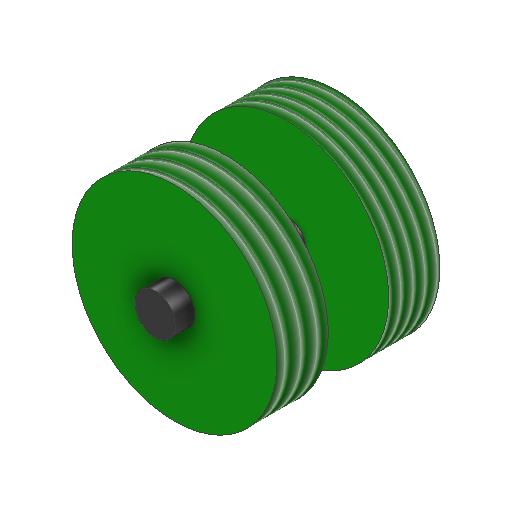
# Autodesk Inventor part: Coletor - Hand
Saved by Autodesk Inventor 2025.3 (Build 293356000, 356)
## iProperties
Created: 2026-05-13
Part Number: Coletor - Hand
Material: Genérico
Document SubType Name: Modeling
Designer: djair.oliveira
Density: 1 g/cm^3
Appearance: Padrão
Author: djair.oliveira
Autodesk Inventor part; units mm, degrees
ref_plane "YZ Plane" through (0, 0, 0) normal (1, 0, 0) x (0, 1, 0)
ref_plane "XZ Plane" through (0, 0, 0) normal (0, 1, 0) x (-1, 0, 0)
ref_plane "XY Plane" through (0, 0, 0) normal (0, 0, 1) x (1, 0, 0)
sketch "Esboço1" plane through (0, 0, 0) normal (1, 0, 0) x (0, 1, 0)
  line L0 (0, 0) -> (0, 100)
  line L1 (0, 100) -> (10, 100)
  line L2 (10, 100) -> (10, 90.4)
  line L3 (10, 90.4) -> (50.8, 90.4)
  line L4 (50.8, 90.4) -> (50.8, 65)
  line L5 (50.8, 65) -> (10, 65)
  line L6 (10, 65) -> (10, 35)
  line L7 (10, 35) -> (50.8, 35)
  line L8 (50.8, 35) -> (50.8, 9.6)
  line L9 (50.8, 9.6) -> (10, 9.6)
  line L10 (10, 9.6) -> (10, 0)
  line L11 (10, 0) -> (0, 0)
  line L12 (0, 50) -> (10, 50)
  dimension "d0" = 10
  dimension "d1" = 100
  dimension "d2" = 25.4
  dimension "d3" = 25.4
  dimension "d4" = 15
  dimension "d5" = 15
  dimension "d6" = 50.8
  constraints: 26 end point, 8 perpendicular, 6 point on line, 2 midpoint, 1 horizontal, 1 vertical
  measures "d0" distance of L10.end L0.start
  measures "d1" distance of L0.start L0.end
  measures "d2" distance of L3.end L4.end
  measures "d3" distance of L7.end L8.end
  measures "d4" distance between parallel lines of L5 L12
  measures "d5" distance between parallel lines of L12 L7
  measures "d6" distance between parallel lines of L0 L4
revolve "Revolução1" add sketch "Esboço1" angle 360 about axis through (0, 0, 0) along (0, 0, 1)
thread "Rosca1" size "M1060x8" class "6g" standard "ANSI Metric M Profile" full length
thread "Rosca2" size "M105x6" class "6g" standard "ANSI Metric M Profile" full length
equation "\"d3\" = d2"
equation "\"d5\" = d4"
